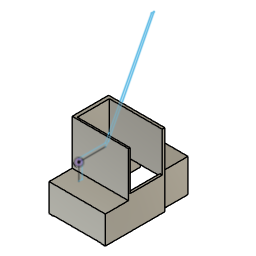
houder_yod_recoder v1 (Autodesk Fusion 360 design; units mm, degrees)
Autodesk Fusion 360 part; units mm, degrees
note: some values were not read from the file. Chosen so that the rebuilt part matches the saved one: which face or edge a step refers to; which pieces of a blend or face edit are solid.
sketch "Sketch1" plane through (0, 0, 0) normal (1, 0, 0) x (0, 1, 0)
  line L0 (0, 0) -> (0, 5)
  line L1 (0, 5) -> (40, 5)
  line L2 (40, 5) -> (110, 140)
  line L3 (110, 140) -> (113.6124, 140)
  line L4 (113.6124, 140) -> (45, 5)
  line L5 (45, 5) -> (40, 0)
  line L6 (40, 0) -> (0, 0)
  constraint coincident L0.start L6.end
  constraint vertical L0
  constraint perpendicular L0 L1
  constraint horizontal L3
  constraint perpendicular L0 L6
extrude "Extrude1" add sketch "Sketch1" along normal blind 75 makes body 1
sketch "Sketch2" plane through (0, 0, 0) normal (1, 0, 0) x (0, 1, 0)
  line L0 (85, 85, 65) -> (85, 0, 65)
  line L1 (85, 0, 65) -> (89, 0, 65)
  line L2 (89, 0, 65) -> (88, 90, 65)
  line L3 (88, 90, 65) -> (85, 85, 65)
sketch "Sketch3" plane through (0, 0, 0) normal (1, 0, 0) x (0, 1, 0)
  line L0 (89, 0, 35) -> (88, 90, 35)
  line L1 (85, 85, 35) -> (85, 0, 35)
  line L2 (89, 0, 35) -> (85, 0, 35)
  line L3 (88, 90, 35) -> (85, 85, 35)
sketch "Sketch3 (curves 35 mm off its plane)" plane through (35, 0, 0) normal (1, 0, 0) x (0, 1, 0)
  line L0 (89, 0) -> (88, 90)
  line L1 (85, 85) -> (85, 0)
  line L2 (89, 0) -> (85, 0)
  line L3 (88, 90) -> (85, 85)
extrude "Extrude2" add sketch "Sketch3 (curves 35 mm off its plane)" along normal blind 5 separate body makes body 2
sketch "Sketch2 (curves 65 mm off its plane)" plane through (65, 0, 0) normal (1, 0, 0) x (0, 1, 0)
  line L0 (85, 85) -> (85, 0)
  line L1 (85, 0) -> (89, 0)
  line L2 (89, 0) -> (88, 90)
  line L3 (88, 90) -> (85, 85)
extrude "Extrude3" add sketch "Sketch2 (curves 65 mm off its plane)" against normal blind 5 separate body makes body 3
move_body "Move1" bodies 2 to x (1, 0, 0) y (0, 1, 0) z (0, 0, 1) at (-20, 0, 0)
extrude "Extrude4" add 1 faces at (63.3333, 86.3333, 0) along direction (0, 0, -1) blind 25 on bodies 3 bodies 3
extrude "Extrude5" add 1 faces at (16.6667, 87.6667, 0) along direction (0, 0, -1) blind 25 on bodies 2 bodies 2
sketch "Sketch4" plane through (0, 0, 0) normal (1, 0, 0) x (0, 1, 0)
  line L0 (0, 0) -> (5, 0)
  line L1 (5, 0) -> (5, -25)
  line L2 (5, -25) -> (0, -25)
  line L3 (0, -25) -> (0, 0)
  constraint horizontal L0
  constraint vertical L1
  constraint horizontal L2
  constraint vertical L3
  constraint coincident L0.start L3.end
extrude "Extrude6" add sketch "Sketch4" along normal blind 75 bodies 1
sketch "Sketch5" plane through (0, 0, 0) normal (1, 0, 0) x (0, 1, 0)
  line L0 (0, -25) -> (90, -25)
  line L1 (90, -25) -> (90, 0)
  line L2 (90, 0) -> (0, 0)
  line L3 (0, 0) -> (0, -25)
  line L4 (90, 0) -> (0, 0)
  line L5 (0, -25) -> (90, -25)
  line L6 (90, -25, 75) -> (90, 0, 75)
  line L7 (0, 0, 75) -> (0, -25, 75)
  line L8 (0, -25, 75) -> (90, -25, 75)
  line L9 (90, 0, 75) -> (0, 0, 75)
  constraint horizontal L0
  constraint vertical L1
  constraint horizontal L2
  constraint vertical L3
  constraint horizontal L5
  constraint horizontal L4
sketch "Sketch5 (curves 75 mm off its plane)" plane through (75, 0, 0) normal (1, 0, 0) x (0, 1, 0)
  line L0 (90, -25) -> (90, 0)
  line L1 (0, 0) -> (0, -25)
  line L2 (0, -25) -> (90, -25)
  line L3 (90, 0) -> (0, 0)
extrude "Extrude7" add sketch "Sketch5 (curves 75 mm off its plane)" against normal blind 3 bodies 1
extrude "Extrude8" add sketch "Sketch5" along normal blind 3 bodies 1
sketch "Sketch6" plane through (0, 0, 0) normal (0, 1, 0) x (1, 0, 0)
  line L0 (2.0876, -1.927) -> (73.2252, -1.927)
  line L1 (73.2252, -1.927) -> (73.2252, 49.2843)
  line L2 (73.2252, 49.2843) -> (2.0876, 49.2843)
  line L3 (2.0876, 49.2843) -> (2.0876, -1.927)
  constraint horizontal L0
  constraint vertical L1
  constraint horizontal L2
  constraint vertical L3
sketch "Sketch7" plane through (0, 0, 5) normal (0, 0, 1) x (-1, 0, 0)
  line L0 (0, -40) -> (0, 0)
  line L1 (0, 0) -> (-75, 0)
  line L2 (-75, 0) -> (-75, -40)
  line L3 (-75, -40) -> (0, -40)
  line L4 (-3.0511, -37.0944) -> (-73.3858, -37.0944)
  line L5 (-73.3858, -37.0944) -> (-73.3858, -2.5693)
  line L6 (-73.3858, -2.5693) -> (-3.0511, -2.5693)
  line L7 (-3.0511, -2.5693) -> (-3.0511, -37.0944)
  constraint horizontal L4
  constraint vertical L5
  constraint horizontal L6
  constraint vertical L7
extrude "Extrude9" cut sketch "Sketch7" against normal blind 5 contours L4 L5 L6 L7 bodies 1
sketch "Sketch8" plane through (0, 0, 0) normal (0, 0, 1) x (1, 0, 0)
  line L0 (75, 0) -> (0, 0)
  line L1 (0, 0) -> (0, 5)
  line L2 (0, 5) -> (75, 5)
  line L3 (75, 5) -> (75, 0)
  constraint horizontal L0
  constraint vertical L1
  constraint horizontal L2
  constraint vertical L3
extrude "Extrude10" add sketch "Sketch8" against normal blind 10 bodies 1
sketch "Sketch9" plane through (0, 0, 0) normal (0, 0, 1) x (1, 0, 0)
  line L0 (0, 40) -> (75, 40)
  line L1 (75, 40) -> (75, 90)
  line L2 (75, 90) -> (0, 90)
  line L3 (0, 90) -> (0, 40)
  constraint horizontal L0
  constraint vertical L1
  constraint horizontal L2
  constraint vertical L3
extrude "Extrude11" add sketch "Sketch9" against normal blind 3 bodies 1 2 3
delete_face "DeleteFace1" 1 faces at (25, 63.3333, 50) on bodies 1
sketch "Sketch10" plane through (0, 0, 0) normal (0, 0, 1) x (1, 0, 0)
  line L0 (-5, 50) -> (85, 50)
  line L1 (85, 50) -> (85, -5)
  line L2 (85, -5) -> (-5, -5)
  line L3 (-5, -5) -> (-5, 50)
  constraint horizontal L0
  constraint vertical L1
  constraint horizontal L2
  constraint vertical L3
extrude "Extrude12" add sketch "Sketch10" along normal blind 70 bodies 1
extrude "Extrude13" cut 1 faces at (25, 31.6667, 70) along direction (0, 0, -1) blind 30 on bodies 1 bodies 1
sketch "Sketch11" plane through (0, 0, 5) normal (0, 0, 1) x (-1, 0, 0)
extrude "Extrude14" add sketch "Sketch7" along normal blind 50 separate body contours L4 L5 L6 L7 makes body 4
move_body "Move2" bodies 4 to x (1, 0, 0) y (0, 1, 0) z (0, 0, 1) at (0, 0, -20)
extrude "Extrude15" add 1 faces at (26.496, 25.586, 35) along direction (0, 0, 1) blind 20 on bodies 4 bodies 4
move_face "OffsetFaces1" offset 50 1 faces at (26.496, 25.586, -15) on bodies 4
move_face "OffsetFaces2" offset 5 1 faces at (49.9409, 2.5693, 15) on bodies 4
move_face "OffsetFaces3" offset 5 1 faces at (26.496, 37.0944, 15) on bodies 4
move_face "OffsetFaces4" offset 3 1 faces at (73.3858, 27.2527, -25) on bodies 4
move_face "OffsetFaces5" offset 3 1 faces at (3.0511, 12.411, -25) on bodies 4
combine "Combine1" operation cut target body 1 tool bodies 4
extrude "Extrude16" add sketch "Sketch6" against normal blind 5 bodies 1
move_face "OffsetFaces6" offset 50 1 faces at (-3.3333, 15, 0) on bodies 1
extrude "Extrude17" add 1 faces at (82.1286, 29.0315, 0) along direction (0, 0, -1) blind 25 on bodies 1 bodies 1
move_face "OffsetFaces7" offset -5 1 faces at (85, 13.3333, -3.3333) on bodies 1
move_face "OffsetFaces8" offset 25 1 faces at (77.1286, 47.3648, -25) on bodies 1
move_face "OffsetFaces9" offset 25 1 faces at (2, 60.6981, -25) on bodies 1
delete_face "DeleteFace2" 1 faces at (16.6667, 89, -10.3333) on bodies 1
delete_face "DeleteFace3" 5 faces at (65, 86.3333, -17.6667) (63.3333, 85, -10.3333) (63.3333, 89, -10.3333) (60, 86.3333, -17.6667) (63.3333, 86.3333, -25) on bodies 1
delete_face "DeleteFace4" 1 faces at (63.3333, 88.9815, 1.6667) on bodies 1
delete_face "DeleteFace5" 5 faces at (20, 87.6481, 1.6667) (16.6667, 88.9815, 1.6667) (16.6667, 85, 3.3333) (15, 87.6481, 1.6667) (16.6667, 87.6296, 5) on bodies 1
sketch "Sketch12" plane through (0, 42.0944, 0) normal (0, -1, 0) x (1, 0, 0)
  line L0 (76.3858, 40) -> (0.0511, 40)
  line L1 (0.0511, 40) -> (0.0511, -50)
  line L2 (0.0511, -50) -> (3, -50)
  line L3 (3, -50) -> (3, -3)
  line L4 (3, -3) -> (72, -3)
  line L5 (72, -3) -> (72, -50)
  line L6 (72, -50) -> (76.3858, -50)
  line L7 (76.3858, -50) -> (76.3858, 40)
  line L8 (3, -3) -> (72, -3)
  line L9 (72, -3) -> (72, -26.5)
  line L10 (72, -26.5) -> (3, -26.5)
  line L11 (3, -26.5) -> (3, -3)
  constraint horizontal L8
  constraint vertical L9
  constraint horizontal L10
  constraint vertical L11
  constraint midpoint L5 L9.end
  constraint coincident L3.end L4.start
extrude "Extrude18" add sketch "Sketch12" against normal blind 3 separate body contours L3 L4 L5 L8 L9 L10 L11 makes body 5
move_face "OffsetFaces10" offset 2 1 faces at (49, 42.0944, -18.6667) on bodies 5
combine "Combine2" operation add target body 1 tool bodies 5
sketch "Sketch13" plane through (0.0511, 0, 0) normal (1, 0, 0) x (0, 1, 0)
  line L0 (-2.4307, -50) -> (42.0944, -50)
  line L1 (42.0944, -50) -> (42.0944, 40)
  line L2 (42.0944, 40) -> (-2.4307, 40)
  line L3 (-2.4307, 40) -> (-2.4307, -50)
  line L4 (-2.4307, 40) -> (48, 40)
  line L5 (48, 40) -> (48, 0)
  line L6 (48, 0) -> (-2.4307, 0)
  line L7 (-2.4307, 0) -> (-2.4307, 40)
  constraint horizontal L4
  constraint vertical L5
  constraint horizontal L6
  constraint vertical L7
  constraint coincident L2.end L3.start
extrude "Extrude19" cut sketch "Sketch13" along normal blind 122 contours L1 L2 L3 L4 L6 L7 bodies 1
move_face "OffsetFaces11" offset -4 1 faces at (50.6837, 42.0944, 25.6667) on bodies 1
extrude "Extrude20" cut 1 faces at (49, 40.0944, -18.6667) along direction (0, 1, 0) blind 8 on bodies 1 bodies 1
move_face "MoveFace1" by (0, -60.6835, 0) 1 faces at (75, 76.6667, -16.6667) on bodies 1
sketch "Sketch14" plane through (0, -5, 0) normal (0, -1, 0) x (1, 0, 0)
  line L0 (80, -50) -> (80, 40)
  line L1 (80, 40) -> (-5, 40)
  line L2 (-5, 40) -> (-5, -50)
  line L3 (-5, -50) -> (2.0876, -50)
  line L4 (2.0876, -50) -> (2.0876, -49.2843)
  line L5 (2.0876, -49.2843) -> (73.2252, -49.2843)
  line L6 (73.2252, -49.2843) -> (73.2252, -50)
  line L7 (73.2252, -50) -> (80, -50)
  line L8 (-5, -50) -> (80, -50)
  line L9 (80, -50) -> (80, -8)
  line L10 (80, -8) -> (-5, -8)
  line L11 (-5, -8) -> (-5, -50)
  constraint horizontal L8
  constraint vertical L9
  constraint horizontal L10
  constraint vertical L11
  constraint coincident L0 L9.end
  constraint coincident L2.end L3.start
extrude "Extrude21" add sketch "Sketch14" along normal blind 35 contours L0 L2 L3 L4 L5 L6 L7 L8 L9 L10 L11 bodies 1
sketch "Sketch15" plane through (0, 0, 0) normal (0, 0, 1) x (1, 0, 0)
sketch "Sketch16" plane through (0, 0, 0) normal (0, 1, 0) x (-1, 0, 0)
  line L0 (-2.0876, 0) -> (-73.2252, 0)
  line L1 (-73.2252, 0) -> (-73.2252, -49.2843)
  line L2 (-73.2252, -49.2843) -> (-2.0876, -49.2843)
  line L3 (-2.0876, -49.2843) -> (-2.0876, 0)
  line L4 (-73.2252, -49.2843) -> (-3.3289, -49.2843)
  line L5 (-3.3289, -49.2843) -> (-3.3289, -17.074)
  line L6 (-3.3289, -17.074) -> (-73.2252, -17.074)
  line L7 (-73.2252, -17.074) -> (-73.2252, -49.2843)
  constraint horizontal L4
  constraint vertical L5
  constraint horizontal L6
  constraint vertical L7
  constraint coincident L1.end L2.start
extrude "Extrude22" cut sketch "Sketch16" against normal blind 35 contours L1 L2 L4 L5 L6 L7 bodies 1
move_face "MoveFace2" by (0, 0, 20) 1 faces at (-3.3163, 30.3648, 40) on bodies 1
